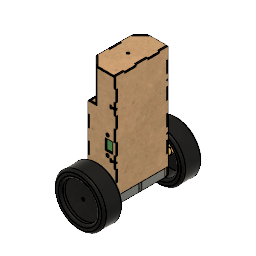
yabr6 (Autodesk Fusion 360 design; units mm, degrees)
Autodesk Fusion 360 part; units mm, degrees
note: some values were not read from the file. Chosen so that the rebuilt part matches the saved one: which bodies a step acts on. Set by a fixed rule: which sketch regions a step uses.
sketch "Sketch1" plane through (0, 0, 0) normal (0, 0, 1) x (1, 0, 0) in component "Steppers"
  line L0 (-16.6565, 21.25) -> (16.6565, 21.25)
  line L1 (21.25, 16.6565) -> (21.25, -16.6565)
  line L2 (16.6565, -21.25) -> (-16.6565, -21.25)
  line L3 (-21.25, -16.6565) -> (-21.25, 16.6565)
  circle A0 centre (-15.5, 15.5) radius 1.5
  circle A1 centre (15.5, 15.5) radius 1.5
  circle A2 centre (15.5, -15.5) radius 1.5
  circle A3 centre (-15.5, -15.5) radius 1.5
  circle A4 centre (0, 0) radius 2.5
  circle A5 centre (0, 0) radius 11.25
  arc A6 (-16.6565, 21.25) -> (-21.25, 16.6565) centre (0, 0) ccw
  arc A7 (-21.25, -16.6565) -> (-16.6565, -21.25) centre (0, 0) ccw
  arc A8 (16.6565, -21.25) -> (21.25, -16.6565) centre (0, 0) ccw
  arc A9 (21.25, 16.6565) -> (16.6565, 21.25) centre (0, 0) ccw
  dimension "d3" = 21.25
  dimension "d4" = 21.25
  dimension "d5" = 3
  dimension "d6" = 3
  dimension "d7" = 3
  dimension "d8" = 3
  dimension "d9" = 15.5
  dimension "d10" = 15.5
  dimension "d11" = 15.5
  dimension "d12" = 15.5
  dimension "d13" = 15.5
  dimension "d14" = 15.5
  dimension "d15" = 15.5
  dimension "d16" = 15.5
  dimension "d17" = 5
  dimension "d18" = 22.5
  dimension "d28" = 42.5
  dimension "d29" = 42.5
  dimension "d30" = 27
  dimension "d31" = 27
  dimension "d32" = 27
  dimension "d33" = 27
  measures "d3" distance of A4.centre L3
  measures "d4" distance of A4.centre L0
  measures "d5" diameter of A0
  measures "d6" diameter of A1
  measures "d7" diameter of A2
  measures "d8" diameter of A3
  measures "d9" distance of A4.centre
  measures "d10" distance of A4.centre
  measures "d11" distance of A4.centre
  measures "d12" distance of A4.centre
  measures "d13" distance of A4.centre
  measures "d14" distance of A4.centre
  measures "d15" distance of A4.centre
  measures "d16" distance of A4.centre
  measures "d17" diameter of A4
  measures "d18" diameter of A5
  measures "d28" distance of L1 L3
  measures "d29" distance of L0 L2
  measures "d30" radius of A6
  measures "d31" radius of A7
  measures "d32" radius of A8
  measures "d33" radius of A9
extrude "Extrude1" add sketch "Sketch1" along normal mid plane 85 contours L0 L1 L2 L3 A6 A7 A8 A9 | A4 | A5 makes body 1 in component "Steppers"
extrude "Extrude2" add sketch "Sketch1" along normal mid plane 90 contours A4 | A5 bodies 1 in component "Steppers"
extrude "Extrude3" add sketch "Sketch1" along normal mid plane 134 contours A4 bodies 1 in component "Steppers"
extrude "Extrude4" cut sketch "Sketch1" along normal mid plane 5 contours L0 L1 L2 L3 A6 A7 A8 A9 | A0 | A1 | A2 | A3 | A4 | A5 bodies 1 makes body 2 at (4.8001, -4.8266, 2.5) in component "Steppers"
sketch "Sketch1 (2)" plane through (0, 0, 42.5) normal (0, 0, 1) x (1, 0, 0) in component "MDF"
  circle A0 centre (0, 0) radius 11.25
  circle A1 centre (-15.5, -15.5) radius 1.5
  circle A2 centre (15.5, -15.5) radius 1.5
  circle A3 centre (15.5, 15.5) radius 1.5
  circle A4 centre (-15.5, 15.5) radius 1.5
  arc A5 (16.6565, -21.25) -> (21.25, -16.6565) centre (0, 0) ccw
  line L0 (21.25, -16.6565) -> (21.25, 16.6565)
  arc A6 (21.25, 16.6565) -> (16.6565, 21.25) centre (0, 0) ccw
  line L1 (16.6565, 21.25) -> (-16.6565, 21.25)
  arc A7 (-16.6565, 21.25) -> (-21.25, 16.6565) centre (0, 0) ccw
  line L2 (-21.25, 16.6565) -> (-21.25, -16.6565)
  arc A8 (-21.25, -16.6565) -> (-16.6565, -21.25) centre (0, 0) ccw
  line L3 (-16.6565, -21.25) -> (16.6565, -21.25)
  line L4 (-24.25, -11.8717) -> (-24.25, 120)
  line L5 (-24.25, 120) -> (24.25, 120)
  line L6 (24.25, 120) -> (24.25, -11.8717)
  arc A9 (-24.25, -11.8717) -> (24.25, -11.8717) centre (0, 0) ccw
  dimension "d37" = 120
  dimension "d38" = 3
  dimension "d39" = 3
  dimension "d41" = 27
  measures "d38" distance of L2 L4
  measures "d39" distance of L0 L6
  measures "d41" radius of A9
extrude "Extrude1'" add sketch "Sketch1 (2)" along normal blind 3 separate body makes body 3 in component "MDF"
copy_body "CopyPasteBodies1" bodies 3 makes body 4 in component "MDF"
move_body "Move1" bodies 4 to x (1, 0, 0) y (0, 1, 0) z (0, 0, 1) at (0, 0, -88) in component "MDF"
sketch "Sketch1 (3)" plane through (0, 0, 45) normal (0, 0, 1) x (1, 0, 0) in component "Wheels"
  circle A0 centre (0, 0) radius 2.5
  circle A1 centre (0, 0) radius 11.25
  circle A2 centre (0, 0) radius 5.5
  dimension "d47" = 11
  measures "d47" diameter of A2
extrude "Extrude1''" add sketch "Sketch1 (3)" along normal blind 24 from surface at 0.5 separate body contours A2 makes body 5 in component "Wheels"
sketch "Sketch2" plane through (0, 0, 69.5) normal (0, 0, 1) x (1, 0, 0) in component "Wheels"
  circle A0 centre (0, 0) radius 2.5
  circle A1 centre (0, 0) radius 5.5
  line L0 (-3.4641, 6) -> (-6.9282, 0)
  line L1 (-6.9282, 0) -> (-3.4641, -6)
  line L2 (-3.4641, -6) -> (3.4641, -6)
  line L3 (3.4641, -6) -> (6.9282, 0)
  line L4 (6.9282, 0) -> (3.4641, 6)
  line L5 (3.4641, 6) -> (-3.4641, 6)
  dimension "d52" = 6
  measures "d52" distance of A0.centre L5
extrude "Extrude2'" add sketch "Sketch2" along normal blind 6 contours A1 | L0 L1 L2 L3 L4 L5 bodies 5 in component "Wheels"
sketch "Sketch3" plane through (0, 0, 75.5) normal (0, 0, 1) x (1, 0, 0) in component "Wheels"
  circle A0 centre (0, 0) radius 2.5
  line L0 (3.4641, 6) -> (-3.4641, 6)
  line L1 (-3.4641, 6) -> (-6.9282, 0)
  line L2 (-6.9282, 0) -> (-3.4641, -6)
  line L3 (-3.4641, -6) -> (3.4641, -6)
  line L4 (3.4641, -6) -> (6.9282, 0)
  line L5 (6.9282, 0) -> (3.4641, 6)
  circle A1 centre (0, 0) radius 44
  dimension "d56" = 88
  measures "d56" diameter of A1
extrude "Extrude3'" add sketch "Sketch3" along normal blind 2 separate body contours L0 L1 L2 L3 L4 L5 | A1 makes body 6 in component "Wheels"
sketch "Sketch4" plane through (0, 0, 77.5) normal (0, 0, 1) x (1, 0, 0) in component "Wheels"
  circle A0 centre (0, 0) radius 2.5
  circle A1 centre (0, 0) radius 44
  circle A2 centre (0, 0) radius 31
  dimension "d61" = 62
  measures "d61" diameter of A2
extrude "Extrude4'" add sketch "Sketch4" along normal blind 8 and the other way blind 26 contours A1 bodies 6 in component "Wheels"
fillet "Fillet1" radius 4 4 edges at (-28.9021, 11.2101, 85.5) (-41.0224, -15.9111, 85.5) (-41.0224, 15.9111, 51.5) (-28.9021, -11.2101, 51.5) on bodies 6 in component "Wheels"
copy_body "CopyPasteBodies1'" bodies 5 6 makes body 7 makes body 8 in component "Wheels"
move_body "Move1'" bodies 7 8 to x (-1, 0, 0) y (0, 1, 0) z (0, 0, -1) at (0, 0, 0) in component "Wheels"
sketch "Sketch2 (2)" plane through (24.25, 0, 0) normal (1, 0, 0) x (0, 0, -1) in component "MDF"
  line L0 (0, 0) -> (-45.5, 0)
  line L1 (0, 0) -> (45.5, 0)
  line L2 (-45.5, 60) -> (-42.5, 60)
  line L3 (-42.5, 60) -> (-42.5, 80)
  line L4 (-42.5, 80) -> (-45.5, 80)
  line L5 (-45.5, 80) -> (-45.5, 100)
  line L6 (-45.5, 100) -> (-42.5, 100)
  line L7 (-42.5, 100) -> (-42.5, 120)
  line L8 (-42.5, 120) -> (-45.5, 120)
  line L9 (-45.5, 120) -> (-45.5, 140)
  line L10 (-45.5, 140) -> (-42.5, 140)
  line L11 (-42.5, 140) -> (-42.5, 160)
  line L12 (-42.5, 160) -> (-45.5, 160)
  line L13 (-45.5, 160) -> (-45.5, 180)
  line L14 (45.5, 180) -> (45.5, 160)
  line L15 (45.5, 160) -> (42.5, 160)
  line L16 (42.5, 160) -> (42.5, 140)
  line L17 (42.5, 140) -> (45.5, 140)
  line L18 (45.5, 140) -> (45.5, 120)
  line L19 (45.5, 120) -> (42.5, 120)
  line L20 (42.5, 120) -> (42.5, 100)
  line L21 (42.5, 100) -> (45.5, 100)
  line L22 (45.5, 100) -> (45.5, 80)
  line L23 (45.5, 80) -> (42.5, 80)
  line L24 (42.5, 80) -> (42.5, 60)
  line L25 (42.5, 60) -> (45.5, 60)
  line L26 (45.5, 180) -> (30, 180)
  line L27 (30, 180) -> (30, 177)
  line L28 (30, 177) -> (10, 177)
  line L29 (10, 177) -> (10, 180)
  line L30 (10, 180) -> (-10, 180)
  line L31 (-10, 180) -> (-10, 177)
  line L32 (-10, 177) -> (-30, 177)
  line L33 (-30, 177) -> (-30, 180)
  line L34 (-30, 180) -> (-45.5, 180)
  line L35 (0, 0) -> (0, 242.7962) construction
  line L36 (45.5, 60) -> (45.5, 40)
  line L37 (45.5, 40) -> (42.5, 40)
  line L38 (42.5, 40) -> (42.5, 20)
  line L39 (42.5, 20) -> (45.5, 20)
  line L40 (45.5, 20) -> (45.5, 0)
  line L41 (-45.5, 60) -> (-45.5, 40)
  line L42 (-45.5, 40) -> (-42.5, 40)
  line L43 (-42.5, 40) -> (-42.5, 20)
  line L44 (-42.5, 20) -> (-45.5, 20)
  line L45 (-45.5, 20) -> (-45.5, 0)
  dimension "d69" = 3
  dimension "d70" = 20
  dimension "d71" = 3
  dimension "d72" = 20
  dimension "d73" = 3
  dimension "d74" = 20
  dimension "d75" = 3
  dimension "d76" = 20
  dimension "d77" = 3
  dimension "d78" = 20
  dimension "d79" = 3
  dimension "d80" = 20
  dimension "d82" = 3
  dimension "d83" = 20
  dimension "d84" = 3
  dimension "d85" = 20
  dimension "d86" = 3
  dimension "d87" = 20
  dimension "d88" = 3
  dimension "d89" = 20
  dimension "d90" = 3
  dimension "d91" = 20
  dimension "d92" = 3
  dimension "d96" = 20
  dimension "d97" = 10
  dimension "d98" = 10
  dimension "d99" = 3
  dimension "d100" = 20
  dimension "d101" = 3
  dimension "d102" = 3
  dimension "d103" = 20
  dimension "d104" = 3
  dimension "d105" = 3
  dimension "d106" = 20
  dimension "d107" = 20
  dimension "d108" = 20
  dimension "d109" = 3
  dimension "d110" = 3
  dimension "d111" = 20
  dimension "d112" = 20
  dimension "d113" = 20
  measures "d97" distance of L29 L35
  measures "d98" distance of L31 L35
  measures "d100" distance of L0.start
  measures "d103" distance of L0.start
  measures "d106" distance of L0.start
  measures "d111" distance of L0.start
  measures "d112" distance of L0.start
extrude "Extrude2''" add sketch "Sketch2 (2)" against normal blind 3 separate body makes body 9 in component "MDF"
combine "Combine1" operation cut target body 3 tool bodies 9 keep tools in component "MDF"
combine "Combine2" operation cut target body 4 tool bodies 9 keep tools in component "MDF"
sketch "Sketch16" plane through (0, 120, 0) normal (0, 1, 0) x (-1, 0, 0) in component "MDF"
  line L0 (-24.25, -45.5) -> (24.25, -45.5)
  line L1 (24.25, -45.5) -> (24.25, -42.5)
  line L2 (24.25, -42.5) -> (-24.25, -42.5)
  line L3 (-24.25, -42.5) -> (-24.25, -45.5)
  line L4 (24.25, -45.5) -> (-75.4847, -45.5) construction
  line L5 (24.25, -45.5) -> (24.25, 30) construction
  line L6 (24.25, -42.5) -> (-74.737, -42.5) construction
  line L7 (21.25, -45.5) -> (21.25, 30) construction
  line L8 (21.25, -30.2972) -> (9.0472, -42.5)
  line L9 (24.25, -31.5398) -> (10.2898, -45.5)
  line L10 (10.2898, -45.5) -> (8.1685, -43.3787)
  line L11 (9.0472, -42.5) -> (8.1685, -43.3787)
  line L12 (24.25, -31.5398) -> (22.1287, -29.4185)
  line L13 (21.25, -30.2972) -> (22.1287, -29.4185)
  line L14 (8.1685, -43.3787) -> (8.1685, -42.5) construction
  line L15 (22.1287, -29.4185) -> (21.25, -29.4185) construction
  line L16 (0, 0) -> (81.4572, 0) construction
  line L17 (21.25, 30.2972) -> (9.0472, 42.5)
  line L18 (9.0472, 42.5) -> (8.1685, 43.3787)
  line L19 (10.2898, 45.5) -> (8.1685, 43.3787)
  line L20 (24.25, 31.5398) -> (10.2898, 45.5)
  line L21 (24.25, 31.5398) -> (22.1287, 29.4185)
  line L22 (21.25, 30.2972) -> (22.1287, 29.4185)
  dimension "d248" = 3
  dimension "d249" = 3
  dimension "d251" = 45
  dimension "d253" = 3
  dimension "d254" = 18.5
  measures "d248" distance of L4 L6
  measures "d249" distance of L5 L7
  measures "d251" angle of L6 L8
  measures "d253" distance of L8 L9
  measures "d254" distance of L16.start
extrude "Extrude11" add sketch "Sketch16" along normal blind 60 separate body contours L2 L9 L10 L11 | L2 L8 L9 L12 L13 | L17 L18 L19 L20 L21 L22 makes body 10 at (-12.8219, 140, -38.7253) makes body 11 at (-17.4753, 140, 34.0719) in component "MDF"
sketch "Sketch17" plane through (-27.8949, 0, -27.8949) normal (-0.707107, 0, -0.707107) x (-0.707107, 0, 0.707107) in component "MDF"
  line L0 (-24.8973, 120) -> (-5.1547, 120)
  line L1 (-5.1547, 120) -> (-5.1547, 180)
  line L2 (-5.1547, 180) -> (-24.8973, 180)
  line L3 (-24.8973, 180) -> (-24.8973, 120)
  line L4 (-24.8973, 150) -> (-5.1547, 150) construction
  line L5 (-15.026, 180) -> (-15.026, 120) construction
  circle A0 centre (-15.026, 162.7) radius 8.1
  circle A1 centre (-15.026, 137.3) radius 8.1
  dimension "d257" = 12.7
  dimension "d258" = 12.7
  dimension "d259" = 16.2
  dimension "d260" = 16.2
  measures "d257" distance of L4
  measures "d258" distance of L4
  measures "d259" diameter of A0
  measures "d260" diameter of A1
extrude "Extrude12" cut sketch "Sketch17" against normal blind 3 contours A0 | A1 bodies 10 in component "MDF"
sketch "Sketch18" plane through (-27.8949, 0, 27.8949) normal (-0.707107, 0, 0.707107) x (0.707107, 0, 0.707107) in component "MDF"
  line L0 (5.1547, 120) -> (24.8973, 120)
  line L1 (24.8973, 120) -> (24.8973, 180)
  line L2 (24.8973, 180) -> (5.1547, 180)
  line L3 (5.1547, 180) -> (5.1547, 120)
  line L4 (15.026, 180) -> (15.026, 120) construction
  line L5 (24.8973, 150) -> (5.1547, 150) construction
  circle A0 centre (15.026, 162.7) radius 8.1
  circle A1 centre (15.026, 137.3) radius 8.1
  dimension "d263" = 12.7
  dimension "d264" = 12.7
  dimension "d265" = 16.2
  dimension "d266" = 16.2
  measures "d263" distance of L5
  measures "d264" distance of L5
  measures "d265" diameter of A0
  measures "d266" diameter of A1
extrude "Extrude13" cut sketch "Sketch18" against normal blind 3 contours A0 | A1 bodies 11 in component "MDF"
sketch "Sketch19" plane through (-24.25, 0, 0) normal (-1, 0, 0) x (0, 0, 1) in component "MDF"
  line L0 (-45.5, 0) -> (-45.5, 20)
  line L1 (-42.5, 20) -> (-42.5, 40)
  line L2 (-45.5, 40) -> (-45.5, 60)
  line L3 (-42.5, 60) -> (-42.5, 80)
  line L4 (-45.5, 80) -> (-45.5, 100)
  line L5 (-10, 177) -> (-10, 180)
  line L6 (-10, 180) -> (10, 180)
  line L7 (10, 180) -> (10, 177)
  line L8 (10, 177) -> (29.4185, 177)
  line L9 (29.4185, 177) -> (29.4185, 120)
  line L10 (29.4185, 120) -> (42.5, 120)
  line L11 (42.5, 120) -> (42.5, 100)
  line L12 (42.5, 100) -> (45.5, 100)
  line L13 (45.5, 100) -> (45.5, 80)
  line L14 (45.5, 80) -> (42.5, 80)
  line L15 (42.5, 80) -> (42.5, 60)
  line L16 (42.5, 60) -> (45.5, 60)
  line L17 (45.5, 60) -> (45.5, 40)
  line L18 (45.5, 40) -> (42.5, 40)
  line L19 (42.5, 40) -> (42.5, 20)
  line L20 (42.5, 20) -> (45.5, 20)
  line L21 (45.5, 20) -> (45.5, 0)
  line L22 (-45.5, 20) -> (-42.5, 20)
  line L23 (-42.5, 40) -> (-45.5, 40)
  line L24 (-45.5, 60) -> (-42.5, 60)
  line L25 (-42.5, 80) -> (-45.5, 80)
  line L26 (-45.5, 100) -> (-42.5, 100)
  line L27 (-42.5, 100) -> (-42.5, 120)
  line L28 (-42.5, 120) -> (-29.4185, 120)
  line L29 (-29.4185, 120) -> (-29.4185, 177)
  line L30 (-29.4185, 177) -> (-10, 177)
  line L31 (-45.5, 0) -> (45.5, 0)
extrude "Extrude14" add sketch "Sketch19" against normal blind 3 separate body makes body 12 in component "MDF"
combine "Combine5" operation cut target body 4 tool bodies 12 keep tools in component "MDF"
combine "Combine6" operation cut target body 3 tool bodies 12 keep tools in component "MDF"
sketch "Sketch20" plane through (0, 180, 0) normal (0, 1, 0) x (-1, 0, 0) in component "MDF"
  line L0 (-24.25, -10) -> (-21.25, -10)
  line L1 (-21.25, -10) -> (-21.25, 10)
  line L2 (-21.25, 10) -> (-24.25, 10)
  line L3 (-21.25, 45.5) -> (-21.25, 30)
  line L4 (-24.25, 30) -> (-24.25, 10)
  line L5 (-21.25, 10) -> (-21.25, -10)
  line L6 (-24.25, -10) -> (-24.25, -30)
  line L7 (-24.25, -30) -> (-21.25, -30)
  line L8 (-21.25, -45.5) -> (8.1685, -45.5)
  line L9 (8.1685, -45.5) -> (8.1685, -43.3787)
  line L10 (22.1287, -29.4185) -> (8.1685, -43.3787)
  line L11 (8.1685, -43.3787) -> (22.1287, -29.4185)
  line L12 (24.25, -29.4185) -> (24.25, -10)
  line L13 (21.25, -10) -> (21.25, 10)
  line L14 (24.25, 10) -> (24.25, 29.4185)
  line L15 (8.1685, 43.3787) -> (22.1287, 29.4185)
  line L16 (22.1287, 29.4185) -> (8.1685, 43.3787)
  line L17 (8.1685, 43.3787) -> (8.1685, 45.5)
  line L18 (8.1685, 45.5) -> (-21.25, 45.5)
  line L19 (-21.25, -45.5) -> (-21.25, -30)
  line L20 (-21.25, -10) -> (-24.25, -10)
  line L21 (-24.25, 10) -> (-21.25, 10)
  line L22 (-21.25, 30) -> (-24.25, 30)
  line L23 (22.1287, 29.4185) -> (24.25, 29.4185)
  line L24 (24.25, 10) -> (21.25, 10)
  line L25 (24.25, -10) -> (21.25, -10)
  line L26 (24.25, -29.4185) -> (22.1287, -29.4185)
extrude "Extrude15" add sketch "Sketch20" against normal blind 3 separate body makes body 13 in component "MDF"
sketch "Sketch21" plane through (0, 0, -45.5) normal (0, 0, -1) x (-1, 0, 0) in component "MDF"
  circle A0 centre (15.5, 15.5) radius 1.5
  circle A1 centre (-15.5, 15.5) radius 1.5
  circle A2 centre (0, 0) radius 11.25
  circle A3 centre (-15.5, -15.5) radius 1.5
  circle A4 centre (15.5, -15.5) radius 1.5
  line L0 (24.25, 0) -> (21.25, 0)
  line L1 (21.25, 0) -> (21.25, 20)
  line L2 (21.25, 20) -> (24.25, 20)
  line L3 (24.25, 20) -> (24.25, 40)
  line L4 (24.25, 40) -> (21.25, 40)
  line L5 (21.25, 40) -> (21.25, 60)
  line L6 (21.25, 60) -> (24.25, 60)
  line L7 (24.25, 60) -> (24.25, 80)
  line L8 (24.25, 80) -> (21.25, 80)
  line L9 (21.25, 80) -> (21.25, 100)
  line L10 (21.25, 100) -> (24.25, 100)
  line L11 (24.25, 100) -> (24.25, 120)
  line L12 (24.25, 120) -> (-24.25, 120)
  line L13 (-24.25, 120) -> (-24.25, 100)
  line L14 (-24.25, 100) -> (-21.25, 100)
  line L15 (-21.25, 100) -> (-21.25, 80)
  line L16 (-21.25, 80) -> (-24.25, 80)
  line L17 (-24.25, 80) -> (-24.25, 60)
  line L18 (-24.25, 60) -> (-21.25, 60)
  line L19 (-21.25, 60) -> (-21.25, 40)
  line L20 (-21.25, 40) -> (-24.25, 40)
  line L21 (-24.25, 40) -> (-24.25, 20)
  line L22 (-24.25, 20) -> (-21.25, 20)
  line L23 (-21.25, 20) -> (-21.25, 0)
  line L24 (-21.25, 0) -> (-24.25, 0)
  line L25 (-24.25, 0) -> (-24.25, -11.8717)
  arc A5 (-24.25, -11.8717) -> (24.25, -11.8717) centre (0, 0) ccw
  line L26 (24.25, -11.8717) -> (24.25, 0)
  line L27 (-21.25, 120) -> (-21.25, 140)
  line L28 (-21.25, 140) -> (-24.25, 140)
  line L29 (-24.25, 140) -> (-24.25, 160)
  line L30 (-24.25, 160) -> (-21.25, 160)
  line L31 (-21.25, 160) -> (-21.25, 177)
  line L32 (-21.25, 177) -> (8.1685, 177)
  line L33 (8.1685, 177) -> (8.1685, 120)
extrude "Extrude16" add sketch "Sketch21" against normal blind 3 contours L12 L27 L28 L29 L30 L31 L32 L33 bodies 4 in component "MDF"
sketch "Sketch22" plane through (0, 0, 45.5) normal (0, 0, 1) x (1, 0, 0) in component "MDF"
  line L0 (-21.25, 0) -> (-24.25, 0)
  line L1 (-24.25, 0) -> (-24.25, -11.8717)
  arc A0 (-24.25, -11.8717) -> (24.25, -11.8717) centre (0, 0) ccw
  line L2 (24.25, -11.8717) -> (24.25, 0)
  line L3 (24.25, 0) -> (21.25, 0)
  line L4 (21.25, 0) -> (21.25, 20)
  line L5 (21.25, 20) -> (24.25, 20)
  line L6 (24.25, 20) -> (24.25, 40)
  line L7 (24.25, 40) -> (21.25, 40)
  line L8 (21.25, 40) -> (21.25, 60)
  line L9 (21.25, 60) -> (24.25, 60)
  line L10 (24.25, 60) -> (24.25, 80)
  line L11 (24.25, 80) -> (21.25, 80)
  line L12 (21.25, 80) -> (21.25, 100)
  line L13 (21.25, 100) -> (24.25, 100)
  line L14 (24.25, 100) -> (24.25, 120)
  line L15 (24.25, 120) -> (-24.25, 120)
  line L16 (-24.25, 120) -> (-24.25, 100)
  line L17 (-24.25, 100) -> (-21.25, 100)
  line L18 (-21.25, 100) -> (-21.25, 80)
  line L19 (-21.25, 80) -> (-24.25, 80)
  line L20 (-24.25, 80) -> (-24.25, 60)
  line L21 (-24.25, 60) -> (-21.25, 60)
  line L22 (-21.25, 60) -> (-21.25, 40)
  line L23 (-21.25, 40) -> (-24.25, 40)
  line L24 (-24.25, 40) -> (-24.25, 20)
  line L25 (-24.25, 20) -> (-21.25, 20)
  line L26 (-21.25, 20) -> (-21.25, 0)
  circle A1 centre (-15.5, 15.5) radius 1.5
  circle A2 centre (15.5, 15.5) radius 1.5
  circle A3 centre (0, 0) radius 11.25
  circle A4 centre (15.5, -15.5) radius 1.5
  circle A5 centre (-15.5, -15.5) radius 1.5
  line L27 (21.25, 120) -> (21.25, 140)
  line L28 (21.25, 140) -> (24.25, 140)
  line L29 (24.25, 140) -> (24.25, 160)
  line L30 (24.25, 160) -> (21.25, 160)
  line L31 (21.25, 160) -> (21.25, 177)
  line L32 (21.25, 177) -> (-8.1685, 177)
  line L33 (-8.1685, 177) -> (-8.1685, 120)
extrude "Extrude17" add sketch "Sketch22" against normal blind 3 contours L15 L27 L28 L29 L30 L31 L32 L33 bodies 3 in component "MDF"
sketch "Sketch23" plane through (-24.25, 0, 0) normal (-1, 0, 0) x (0, 0, 1) in component "MDF"
  line L0 (-45.5, 20) -> (-45.5, 0)
  line L1 (-45.5, 0) -> (45.5, 0)
  line L2 (45.5, 0) -> (45.5, 20)
  line L3 (45.5, 20) -> (42.5, 20)
  line L4 (42.5, 20) -> (42.5, 40)
  line L5 (42.5, 40) -> (45.5, 40)
  line L6 (45.5, 40) -> (45.5, 60)
  line L7 (45.5, 60) -> (42.5, 60)
  line L8 (42.5, 60) -> (42.5, 80)
  line L9 (42.5, 80) -> (45.5, 80)
  line L10 (45.5, 80) -> (45.5, 100)
  line L11 (45.5, 100) -> (42.5, 100)
  line L12 (42.5, 100) -> (42.5, 120)
  line L13 (42.5, 120) -> (29.4185, 120)
  line L14 (29.4185, 120) -> (29.4185, 177)
  line L15 (29.4185, 177) -> (10, 177)
  line L16 (10, 177) -> (10, 180)
  line L17 (10, 180) -> (-10, 180)
  line L18 (-10, 180) -> (-10, 177)
  line L19 (-10, 177) -> (-29.4185, 177)
  line L20 (-29.4185, 177) -> (-29.4185, 120)
  line L21 (-29.4185, 120) -> (-42.5, 120)
  line L22 (-42.5, 120) -> (-42.5, 100)
  line L23 (-42.5, 100) -> (-45.5, 100)
  line L24 (-45.5, 100) -> (-45.5, 80)
  line L25 (-45.5, 80) -> (-42.5, 80)
  line L26 (-42.5, 80) -> (-42.5, 60)
  line L27 (-42.5, 60) -> (-45.5, 60)
  line L28 (-45.5, 60) -> (-45.5, 40)
  line L29 (-45.5, 40) -> (-42.5, 40)
  line L30 (-42.5, 40) -> (-42.5, 20)
  line L31 (-42.5, 20) -> (-45.5, 20)
  line L32 (0, 180) -> (0, 120) construction
  line L33 (-29.4185, 120) -> (29.4185, 120) construction
  line L34 (0, 150) -> (20, 150) construction
  line L35 (0, 150) -> (-20, 150) construction
  circle A0 centre (0, 162.7) radius 8.1
  circle A1 centre (0, 137.3) radius 8.1
  dimension "d277" = 12.7
  dimension "d278" = 12.7
  dimension "d279" = 16.2
  dimension "d280" = 16.2
  measures "d278" distance of L34 origin
  measures "d279" diameter of A0
  measures "d280" diameter of A1
extrude "Extrude18" cut sketch "Sketch23" against normal blind 3 contours A0 | A1 bodies 12 in component "MDF"
sketch "Sketch1 (4)" plane through (0, 0, 0) normal (0, 1, 0) x (1, 0, 0) in component "ground plane"
  line L0 (-5000, 5000) -> (5000, 5000)
  line L1 (5000, 5000) -> (5000, -5000)
  line L2 (5000, -5000) -> (-5000, -5000)
  line L3 (-5000, -5000) -> (-5000, 5000)
extrude "Extrude1'''" add sketch "Sketch1 (4)" against normal blind 50 from surface at -44 separate body makes body 14 in component "ground plane"
sketch "Sketch1 (5)" plane through (21.25, 0, 0) normal (-1, 0, 0) x (0, 0, 1) in component "pcb"
  line L0 (45.5, 40) -> (45.5, 60)
  line L1 (45.5, 60) -> (42.5, 60)
  line L2 (42.5, 60) -> (42.5, 80)
  line L3 (42.5, 80) -> (45.5, 80)
  line L4 (45.5, 80) -> (45.5, 100)
  line L5 (45.5, 100) -> (42.5, 100)
  line L6 (42.5, 100) -> (42.5, 120)
  line L7 (42.5, 120) -> (45.5, 120)
  line L8 (45.5, 120) -> (45.5, 140)
  line L9 (45.5, 140) -> (42.5, 140)
  line L10 (42.5, 140) -> (42.5, 160)
  line L11 (42.5, 160) -> (45.5, 160)
  line L12 (45.5, 160) -> (45.5, 180)
  line L13 (45.5, 180) -> (30, 180)
  line L14 (30, 180) -> (30, 177)
  line L15 (30, 177) -> (10, 177)
  line L16 (10, 177) -> (10, 180)
  line L17 (10, 180) -> (-10, 180)
  line L18 (-10, 180) -> (-10, 177)
  line L19 (-10, 177) -> (-30, 177)
  line L20 (-30, 177) -> (-30, 180)
  line L21 (-30, 180) -> (-45.5, 180)
  line L22 (-45.5, 180) -> (-45.5, 160)
  line L23 (-45.5, 160) -> (-42.5, 160)
  line L24 (-42.5, 160) -> (-42.5, 140)
  line L25 (-42.5, 140) -> (-45.5, 140)
  line L26 (-45.5, 140) -> (-45.5, 120)
  line L27 (-45.5, 120) -> (-42.5, 120)
  line L28 (-42.5, 120) -> (-42.5, 100)
  line L29 (-42.5, 100) -> (-45.5, 100)
  line L30 (-45.5, 100) -> (-45.5, 80)
  line L31 (-45.5, 80) -> (-42.5, 80)
  line L32 (-42.5, 80) -> (-42.5, 60)
  line L33 (-42.5, 60) -> (-45.5, 60)
  line L34 (-45.5, 60) -> (-45.5, 40)
  line L35 (-45.5, 40) -> (-42.5, 40)
  line L36 (-42.5, 40) -> (-42.5, 20)
  line L37 (-42.5, 20) -> (-45.5, 20)
  line L38 (-45.5, 20) -> (-45.5, 0)
  line L39 (-45.5, 0) -> (45.5, 0)
  line L40 (45.5, 0) -> (45.5, 20)
  line L41 (45.5, 20) -> (42.5, 20)
  line L42 (42.5, 20) -> (42.5, 40)
  line L43 (42.5, 40) -> (45.5, 40)
  line L44 (-39.37, 26) -> (-39.37, 86.96)
  line L45 (-39.37, 86.96) -> (39.37, 86.96)
  line L46 (39.37, 86.96) -> (39.37, 26)
  line L47 (-39.37, 26) -> (39.37, 26)
  line L48 (-39.37, 56.48) -> (39.37, 56.48) construction
  line L49 (0, 86.96) -> (0, 26) construction
  circle A0 centre (-31.75, 79.34) radius 1.5
  circle A1 centre (31.75, 79.34) radius 1.5
  circle A2 centre (26.67, 38.7) radius 1.5
  circle A3 centre (-26.67, 38.7) radius 1.5
  dimension "d289" = 78.74
  dimension "d290" = 26
  dimension "d291" = 39.37
  dimension "d295" = 3
  dimension "d296" = 3
  dimension "d297" = 3
  dimension "d298" = 3
  dimension "d315" = 12.7
  dimension "d316" = 12.7
  dimension "d317" = 12.7
  dimension "d318" = 12.7
  dimension "d319" = 7.62
  dimension "d320" = 7.62
  dimension "d321" = 60.96
  dimension "d323" = 53.34
  dimension "d324" = 53.34
  measures "d295" diameter of A0
  measures "d296" diameter of A1
  measures "d297" diameter of A3
  measures "d298" diameter of A2
  measures "d321" distance of L45 L47
extrude "Extrude1''''" add sketch "Sketch1 (5)" along normal blind 1 from surface at 40 separate body contours L44 L45 L46 L47 makes body 15 in component "pcb"
sketch "Sketch25" plane through (-18.75, 0, 0) normal (1, 0, 0) x (0, 0, -1) in component "MDF"
  circle A0 centre (-26.67, 38.7) radius 1.5
  circle A1 centre (26.67, 38.7) radius 1.5
  circle A2 centre (-31.75, 79.34) radius 1.5
  circle A3 centre (31.75, 79.34) radius 1.5
  line L0 (39.37, 26) -> (39.37, 86.96)
  line L1 (39.37, 86.96) -> (-39.37, 86.96)
  line L2 (-39.37, 86.96) -> (-39.37, 26)
  line L3 (-39.37, 26) -> (39.37, 26)
extrude "Extrude19" cut sketch "Sketch25" against normal blind 10 contours A0 | A1 | A2 | A3 bodies 12 in component "MDF"
sketch "Sketch1 (6)" plane through (24.25, 0, 0) normal (1, 0, 0) x (0, 0, -1)
  line L0 (-45.5, 60) -> (-45.5, 40)
  line L1 (-45.5, 40) -> (-42.5, 40)
  line L2 (-42.5, 40) -> (-42.5, 20)
  line L3 (-42.5, 20) -> (-45.5, 20)
  line L4 (-45.5, 20) -> (-45.5, 0)
  line L5 (-45.5, 0) -> (45.5, 0)
  line L6 (45.5, 0) -> (45.5, 20)
  line L7 (45.5, 20) -> (42.5, 20)
  line L8 (42.5, 20) -> (42.5, 40)
  line L9 (42.5, 40) -> (45.5, 40)
  line L10 (45.5, 40) -> (45.5, 60)
  line L11 (45.5, 60) -> (42.5, 60)
  line L12 (42.5, 60) -> (42.5, 80)
  line L13 (42.5, 80) -> (45.5, 80)
  line L14 (45.5, 80) -> (45.5, 100)
  line L15 (45.5, 100) -> (42.5, 100)
  line L16 (42.5, 100) -> (42.5, 120)
  line L17 (42.5, 120) -> (45.5, 120)
  line L18 (45.5, 120) -> (45.5, 140)
  line L19 (45.5, 140) -> (42.5, 140)
  line L20 (42.5, 140) -> (42.5, 160)
  line L21 (42.5, 160) -> (45.5, 160)
  line L22 (45.5, 160) -> (45.5, 180)
  line L23 (45.5, 180) -> (30, 180)
  line L24 (30, 180) -> (30, 177)
  line L25 (30, 177) -> (10, 177)
  line L26 (10, 177) -> (10, 180)
  line L27 (10, 180) -> (-10, 180)
  line L28 (-10, 180) -> (-10, 177)
  line L29 (-10, 177) -> (-30, 177)
  line L30 (-30, 177) -> (-30, 180)
  line L31 (-30, 180) -> (-45.5, 180)
  line L32 (-45.5, 180) -> (-45.5, 160)
  line L33 (-45.5, 160) -> (-42.5, 160)
  line L34 (-42.5, 160) -> (-42.5, 140)
  line L35 (-42.5, 140) -> (-45.5, 140)
  line L36 (-45.5, 140) -> (-45.5, 120)
  line L37 (-45.5, 120) -> (-42.5, 120)
  line L38 (-42.5, 120) -> (-42.5, 100)
  line L39 (-42.5, 100) -> (-45.5, 100)
  line L40 (-45.5, 100) -> (-45.5, 80)
  line L41 (-45.5, 80) -> (-42.5, 80)
  line L42 (-42.5, 80) -> (-42.5, 60)
  line L43 (-42.5, 60) -> (-45.5, 60)
  line L44 (-45.5, 60) -> (-42.5, 40) construction
  circle A0 centre (-44, 50) radius 1.5
  line L45 (45.5, 60) -> (42.5, 40) construction
  circle A1 centre (44, 50) radius 1.5
  line L46 (45.5, 140) -> (42.5, 120) construction
  circle A2 centre (44, 130) radius 1.5
  line L47 (-45.5, 140) -> (-42.5, 120) construction
  circle A3 centre (-44, 130) radius 1.5
  dimension "d327" = 3
  dimension "d328" = 3
  dimension "d329" = 3
  dimension "d330" = 3
  measures "d327" diameter of A0
  measures "d328" diameter of A1
  measures "d329" diameter of A2
  measures "d330" diameter of A3
extrude "Extrude20" cut sketch "Sketch1 (6)" against normal blind 3 contours A0 | A1 | A2 | A3 bodies 9 in component "MDF"
sketch "Sketch26" plane through (0, 0, 45.5) normal (0, 0, 1) x (1, 0, 0) in component "MDF"
  line L0 (-21.25, 0) -> (-24.25, 0)
  line L1 (-24.25, 0) -> (-24.25, -11.8717)
  arc A0 (-24.25, -11.8717) -> (24.25, -11.8717) centre (0, 0) ccw
  line L2 (24.25, -11.8717) -> (24.25, 0)
  line L3 (24.25, 0) -> (21.25, 0)
  line L4 (21.25, 0) -> (21.25, 20)
  line L5 (21.25, 20) -> (24.25, 20)
  line L6 (24.25, 20) -> (24.25, 40)
  line L7 (24.25, 40) -> (21.25, 40)
  line L8 (21.25, 40) -> (21.25, 60)
  line L9 (21.25, 60) -> (24.25, 60)
  line L10 (24.25, 60) -> (24.25, 80)
  line L11 (24.25, 80) -> (21.25, 80)
  line L12 (21.25, 80) -> (21.25, 100)
  line L13 (21.25, 100) -> (24.25, 100)
  line L14 (24.25, 100) -> (24.25, 120)
  line L15 (24.25, 120) -> (21.25, 120)
  line L16 (21.25, 120) -> (21.25, 140)
  line L17 (21.25, 140) -> (24.25, 140)
  line L18 (24.25, 140) -> (24.25, 160)
  line L19 (24.25, 160) -> (21.25, 160)
  line L20 (21.25, 160) -> (21.25, 177)
  line L21 (21.25, 177) -> (-8.1685, 177)
  line L22 (-8.1685, 177) -> (-8.1685, 120)
  line L23 (-8.1685, 120) -> (-24.25, 120)
  line L24 (-24.25, 120) -> (-24.25, 100)
  line L25 (-24.25, 100) -> (-21.25, 100)
  line L26 (-21.25, 100) -> (-21.25, 80)
  line L27 (-21.25, 80) -> (-24.25, 80)
  line L28 (-24.25, 80) -> (-24.25, 60)
  line L29 (-24.25, 60) -> (-21.25, 60)
  line L30 (-21.25, 60) -> (-21.25, 40)
  line L31 (-21.25, 40) -> (-24.25, 40)
  line L32 (-24.25, 40) -> (-24.25, 20)
  line L33 (-24.25, 20) -> (-21.25, 20)
  line L34 (-21.25, 20) -> (-21.25, 0)
  circle A1 centre (-15.5, -15.5) radius 1.5
  circle A2 centre (0, 0) radius 11.25
  circle A3 centre (15.5, -15.5) radius 1.5
  circle A4 centre (15.5, 15.5) radius 1.5
  circle A5 centre (-15.5, 15.5) radius 1.5
  line L35 (21.25, 130) -> (21.25, 131.5)
  line L36 (16.75, 131.5) -> (16.75, 132.85)
  line L37 (16.75, 132.85) -> (14.25, 132.85)
  line L38 (14.25, 132.85) -> (14.25, 127.15)
  line L39 (14.25, 127.15) -> (16.75, 127.15)
  line L40 (16.75, 127.15) -> (16.75, 128.5)
  line L41 (16.75, 128.5) -> (21.25, 128.5)
  line L42 (21.25, 130) -> (21.25, 128.5)
  line L43 (21.25, 131.5) -> (16.75, 131.5)
  line L44 (21.25, 50) -> (21.25, 51.5)
  line L45 (21.25, 50) -> (21.25, 48.5)
  line L46 (21.25, 51.5) -> (16.75, 51.5)
  line L47 (16.75, 51.5) -> (16.75, 52.85)
  line L48 (14.25, 47.15) -> (16.75, 47.15)
  line L49 (16.75, 48.5) -> (21.25, 48.5)
  line L50 (16.75, 52.85) -> (14.25, 52.85)
  line L51 (14.25, 52.85) -> (14.25, 47.15)
  line L52 (16.75, 47.15) -> (16.75, 48.5)
  dimension "d333" = 3
  dimension "d334" = 1.5
  dimension "d335" = 2.5
  dimension "d336" = 7
  dimension "d337" = 5.7
  dimension "d338" = 2.85
  dimension "d339" = 3
  dimension "d340" = 1.5
  dimension "d341" = 2.5
  dimension "d342" = 7
  dimension "d343" = 5.7
  dimension "d344" = 2.85
  measures "d333" distance of L41 L43
  measures "d336" distance of L38 A0.centre
  measures "d337" distance of L37 L39
  measures "d338" distance of A0.centre L37
  measures "d339" distance of L46 L49
  measures "d342" distance of A0.centre L51
  measures "d343" distance of L48 L50
  measures "d344" distance of A0.centre L50
extrude "Extrude21" cut sketch "Sketch26" against normal blind 200 contours L8 L44 L45 L46 L47 L48 L49 L50 L51 L52 | L16 L35 L36 L37 L38 L39 L40 L41 L42 L43 bodies 3 4 in component "MDF"
sketch "Sketch27" plane through (0, 180, 0) normal (0, 1, 0) x (-1, 0, 0) in component "MDF"
  line L0 (24.25, -10) -> (21.25, -10)
  line L1 (21.25, -10) -> (21.25, 10)
  line L2 (21.25, 10) -> (24.25, 10)
  line L3 (24.25, 10) -> (24.25, 29.4185)
  line L4 (24.25, 29.4185) -> (22.1287, 29.4185)
  line L5 (22.1287, 29.4185) -> (8.1685, 43.3787)
  line L6 (8.1685, 43.3787) -> (8.1685, 45.5)
  line L7 (8.1685, 45.5) -> (-21.25, 45.5)
  line L8 (-21.25, 45.5) -> (-21.25, 30)
  line L9 (-21.25, 30) -> (-24.25, 30)
  line L10 (-24.25, 30) -> (-24.25, 10)
  line L11 (-24.25, 10) -> (-21.25, 10)
  line L12 (-21.25, 10) -> (-21.25, -10)
  line L13 (-21.25, -10) -> (-24.25, -10)
  line L14 (-24.25, -10) -> (-24.25, -30)
  line L15 (-24.25, -30) -> (-21.25, -30)
  line L16 (-21.25, -30) -> (-21.25, -45.5)
  line L17 (-21.25, -45.5) -> (8.1685, -45.5)
  line L18 (8.1685, -45.5) -> (8.1685, -43.3787)
  line L19 (8.1685, -43.3787) -> (22.1287, -29.4185)
  line L20 (22.1287, -29.4185) -> (24.25, -29.4185)
  line L21 (24.25, -29.4185) -> (24.25, -10)
  circle A0 centre (0, 0) radius 2.5
  dimension "d350" = 5
  measures "d350" diameter of A0
extrude "Extrude23" cut sketch "Sketch27" against normal blind 3 contours A0 bodies 13 in component "MDF"
sketch "Sketch2 (3)" plane through (-21.25, 0, 0) normal (1, 0, 0) x (0, 0, -1)
  circle A0 centre (31.75, 79.34) radius 1.5
  circle A1 centre (26.67, 38.7) radius 1.5
  circle A2 centre (-31.75, 79.34) radius 1.5
  circle A3 centre (-26.67, 38.7) radius 1.5
  circle A4 centre (0, 162.7) radius 8.1
  circle A5 centre (0, 137.3) radius 8.1
  line L0 (45.5, 0) -> (45.5, 20)
  line L1 (45.5, 20) -> (42.5, 20)
  line L2 (42.5, 20) -> (42.5, 40)
  line L3 (42.5, 40) -> (45.5, 40)
  line L4 (45.5, 40) -> (45.5, 60)
  line L5 (45.5, 60) -> (42.5, 60)
  line L6 (42.5, 60) -> (42.5, 80)
  line L7 (42.5, 80) -> (45.5, 80)
  line L8 (45.5, 80) -> (45.5, 100)
  line L9 (45.5, 100) -> (42.5, 100)
  line L10 (42.5, 100) -> (42.5, 120)
  line L11 (42.5, 120) -> (29.4185, 120)
  line L12 (29.4185, 120) -> (29.4185, 177)
  line L13 (29.4185, 177) -> (10, 177)
  line L14 (10, 177) -> (10, 180)
  line L15 (10, 180) -> (-10, 180)
  line L16 (-10, 180) -> (-10, 177)
  line L17 (-10, 177) -> (-29.4185, 177)
  line L18 (-29.4185, 177) -> (-29.4185, 120)
  line L19 (-29.4185, 120) -> (-42.5, 120)
  line L20 (-42.5, 120) -> (-42.5, 100)
  line L21 (-42.5, 100) -> (-45.5, 100)
  line L22 (-45.5, 100) -> (-45.5, 80)
  line L23 (-45.5, 80) -> (-42.5, 80)
  line L24 (-42.5, 80) -> (-42.5, 60)
  line L25 (-42.5, 60) -> (-45.5, 60)
  line L26 (-45.5, 60) -> (-45.5, 40)
  line L27 (-45.5, 40) -> (-42.5, 40)
  line L28 (-42.5, 40) -> (-42.5, 20)
  line L29 (-42.5, 20) -> (-45.5, 20)
  line L30 (-45.5, 20) -> (-45.5, 0)
  line L31 (-45.5, 0) -> (45.5, 0)
  line L32 (-39.37, 86.96) -> (39.37, 86.96)
  line L33 (0, 86.96) -> (-10, 86.96) construction
  line L34 (0, 86.96) -> (10, 86.96) construction
  line L35 (-10, 86.96) -> (-15, 86.96)
  line L36 (-15, 88.46) -> (-10, 88.46)
  line L37 (-10, 88.46) -> (-10, 86.96)
  line L38 (-15, 88.46) -> (-15, 86.96)
  line L39 (10, 86.96) -> (15, 86.96)
  line L40 (15, 86.96) -> (15, 88.46)
  line L41 (15, 88.46) -> (10, 88.46)
  line L42 (10, 88.46) -> (10, 86.96)
  line L43 (-15, 120.96) -> (-10, 120.96)
  line L44 (-10, 120.96) -> (-10, 119.46)
  line L45 (-10, 119.46) -> (-15, 119.46)
  line L46 (-15, 119.46) -> (-15, 120.96)
  line L47 (10, 120.96) -> (15, 120.96)
  line L48 (15, 120.96) -> (15, 119.46)
  line L49 (15, 119.46) -> (10, 119.46)
  line L50 (10, 119.46) -> (10, 120.96)
  dimension "d354" = 10
  dimension "d355" = 5
  dimension "d356" = 1.5
  dimension "d357" = 31
  measures "d354" distance of origin
extrude "Extrude24" cut sketch "Sketch2 (3)" against normal blind 3 contours L32 L35 L36 L37 L38 | L32 L39 L40 L41 L42 | L43 L44 L45 L46 | L47 L48 L49 L50 bodies 12 in component "MDF"
sketch "Sketch3 (2)" plane through (0, 0, 45.5) normal (0, 0, 1) x (1, 0, 0)
  line L0 (16.75, 131.5) -> (21.25, 131.5)
  line L1 (21.25, 131.5) -> (21.25, 140)
  line L2 (21.25, 140) -> (24.25, 140)
  line L3 (24.25, 140) -> (24.25, 160)
  line L4 (24.25, 160) -> (21.25, 160)
  line L5 (21.25, 160) -> (21.25, 177)
  line L6 (21.25, 177) -> (-8.1685, 177)
  line L7 (-8.1685, 177) -> (-8.1685, 120)
  line L8 (-8.1685, 120) -> (-24.25, 120)
  line L9 (-24.25, 120) -> (-24.25, 100)
  line L10 (-24.25, 100) -> (-21.25, 100)
  line L11 (-21.25, 100) -> (-21.25, 80)
  line L12 (-21.25, 80) -> (-24.25, 80)
  line L13 (-24.25, 80) -> (-24.25, 60)
  line L14 (-24.25, 60) -> (-21.25, 60)
  line L15 (-21.25, 60) -> (-21.25, 40)
  line L16 (-21.25, 40) -> (-24.25, 40)
  line L17 (-24.25, 40) -> (-24.25, 20)
  line L18 (-24.25, 20) -> (-21.25, 20)
  line L19 (-21.25, 20) -> (-21.25, 0)
  line L20 (-21.25, 0) -> (-24.25, 0)
  line L21 (-24.25, 0) -> (-24.25, -11.8717)
  arc A0 (-24.25, -11.8717) -> (24.25, -11.8717) centre (0, 0) ccw
  line L22 (24.25, -11.8717) -> (24.25, 0)
  line L23 (24.25, 0) -> (21.25, 0)
  line L24 (21.25, 0) -> (21.25, 20)
  line L25 (21.25, 20) -> (24.25, 20)
  line L26 (24.25, 20) -> (24.25, 40)
  line L27 (24.25, 40) -> (21.25, 40)
  line L28 (21.25, 40) -> (21.25, 48.5)
  line L29 (21.25, 48.5) -> (16.75, 48.5)
  line L30 (16.75, 48.5) -> (16.75, 47.15)
  line L31 (16.75, 47.15) -> (14.25, 47.15)
  line L32 (14.25, 47.15) -> (14.25, 52.85)
  line L33 (14.25, 52.85) -> (16.75, 52.85)
  line L34 (16.75, 52.85) -> (16.75, 51.5)
  line L35 (16.75, 51.5) -> (21.25, 51.5)
  line L36 (21.25, 51.5) -> (21.25, 60)
  line L37 (21.25, 60) -> (24.25, 60)
  line L38 (24.25, 60) -> (24.25, 80)
  line L39 (24.25, 80) -> (21.25, 80)
  line L40 (21.25, 80) -> (21.25, 100)
  line L41 (21.25, 100) -> (24.25, 100)
  line L42 (24.25, 100) -> (24.25, 120)
  line L43 (24.25, 120) -> (21.25, 120)
  line L44 (21.25, 120) -> (21.25, 128.5)
  line L45 (21.25, 128.5) -> (16.75, 128.5)
  line L46 (16.75, 128.5) -> (16.75, 127.15)
  line L47 (16.75, 127.15) -> (14.25, 127.15)
  line L48 (14.25, 127.15) -> (14.25, 132.85)
  line L49 (14.25, 132.85) -> (16.75, 132.85)
  line L50 (16.75, 132.85) -> (16.75, 131.5)
  circle A1 centre (0, 0) radius 11.25
  circle A2 centre (15.5, 15.5) radius 1.5
  circle A3 centre (-15.5, -15.5) radius 1.5
  circle A4 centre (15.5, -15.5) radius 1.5
  circle A5 centre (-15.5, 15.5) radius 1.5
  circle A6 centre (10.25, 54.7) radius 3
  circle A7 centre (10.25, 85.3) radius 3
  line L51 (6.25, 79.3) -> (19.25, 79.3)
  line L52 (19.25, 79.3) -> (19.25, 60.7)
  line L53 (19.25, 60.7) -> (6.25, 60.7)
  line L54 (6.25, 60.7) -> (6.25, 79.3)
  line L55 (19.25, 70) -> (24.25, 70) construction
  line L56 (10.25, 60.7) -> (10.25, 54.7) construction
  line L57 (10.25, 79.3) -> (10.25, 85.3) construction
  dimension "d363" = 6
  dimension "d364" = 6
  dimension "d365" = 18.6
  dimension "d366" = 13
  dimension "d367" = 2
  dimension "d368" = 6
  dimension "d369" = 6
  dimension "d370" = 4
  measures "d363" diameter of A6
  measures "d364" diameter of A7
  measures "d367" distance of A0.centre L52
extrude "Extrude25" cut sketch "Sketch3 (2)" against normal blind 3 contours A6 | A7 | L51 L52 L53 L54 bodies 3 in component "MDF"
sketch "Sketch4 (2)" plane through (0, 0, -42.5) normal (0, 0, 1) x (1, 0, 0)
  line L0 (16.75, 131.5) -> (21.25, 131.5)
  line L1 (21.25, 131.5) -> (21.25, 140)
  line L2 (21.25, 140) -> (24.25, 140)
  line L3 (24.25, 140) -> (24.25, 160)
  line L4 (24.25, 160) -> (21.25, 160)
  line L5 (21.25, 160) -> (21.25, 177)
  line L6 (21.25, 177) -> (-8.1685, 177)
  line L7 (-8.1685, 177) -> (-8.1685, 120)
  line L8 (-8.1685, 120) -> (-24.25, 120)
  line L9 (-24.25, 120) -> (-24.25, 100)
  line L10 (-24.25, 100) -> (-21.25, 100)
  line L11 (-21.25, 100) -> (-21.25, 80)
  line L12 (-21.25, 80) -> (-24.25, 80)
  line L13 (-24.25, 80) -> (-24.25, 60)
  line L14 (-24.25, 60) -> (-21.25, 60)
  line L15 (-21.25, 60) -> (-21.25, 40)
  line L16 (-21.25, 40) -> (-24.25, 40)
  line L17 (-24.25, 40) -> (-24.25, 20)
  line L18 (-24.25, 20) -> (-21.25, 20)
  line L19 (-21.25, 20) -> (-21.25, 0)
  line L20 (-21.25, 0) -> (-24.25, 0)
  line L21 (-24.25, 0) -> (-24.25, -11.8717)
  arc A0 (-24.25, -11.8717) -> (24.25, -11.8717) centre (0, 0) ccw
  line L22 (24.25, -11.8717) -> (24.25, 0)
  line L23 (24.25, 0) -> (21.25, 0)
  line L24 (21.25, 0) -> (21.25, 20)
  line L25 (21.25, 20) -> (24.25, 20)
  line L26 (24.25, 20) -> (24.25, 40)
  line L27 (24.25, 40) -> (21.25, 40)
  line L28 (21.25, 40) -> (21.25, 48.5)
  line L29 (21.25, 48.5) -> (16.75, 48.5)
  line L30 (16.75, 48.5) -> (16.75, 47.15)
  line L31 (16.75, 47.15) -> (14.25, 47.15)
  line L32 (14.25, 47.15) -> (14.25, 52.85)
  line L33 (14.25, 52.85) -> (16.75, 52.85)
  line L34 (16.75, 52.85) -> (16.75, 51.5)
  line L35 (16.75, 51.5) -> (21.25, 51.5)
  line L36 (21.25, 51.5) -> (21.25, 60)
  line L37 (21.25, 60) -> (24.25, 60)
  line L38 (24.25, 60) -> (24.25, 80)
  line L39 (24.25, 80) -> (21.25, 80)
  line L40 (21.25, 80) -> (21.25, 100)
  line L41 (21.25, 100) -> (24.25, 100)
  line L42 (24.25, 100) -> (24.25, 120)
  line L43 (24.25, 120) -> (21.25, 120)
  line L44 (21.25, 120) -> (21.25, 128.5)
  line L45 (21.25, 128.5) -> (16.75, 128.5)
  line L46 (16.75, 128.5) -> (16.75, 127.15)
  line L47 (16.75, 127.15) -> (14.25, 127.15)
  line L48 (14.25, 127.15) -> (14.25, 132.85)
  line L49 (14.25, 132.85) -> (16.75, 132.85)
  line L50 (16.75, 132.85) -> (16.75, 131.5)
  circle A1 centre (-15.5, 15.5) radius 1.5
  circle A2 centre (15.5, -15.5) radius 1.5
  circle A3 centre (-15.5, -15.5) radius 1.5
  circle A4 centre (15.5, 15.5) radius 1.5
  circle A5 centre (0, 0) radius 11.25
  line L51 (9.05, 86.96) -> (17.25, 86.96)
  line L52 (17.25, 86.96) -> (17.25, 68.96)
  line L53 (17.25, 68.96) -> (9.05, 68.96)
  line L54 (9.05, 68.96) -> (9.05, 86.96)
  line L55 (-18.75, 86.96) -> (-9, 86.96) construction
  dimension "d373" = 8.2
  dimension "d374" = 18
  dimension "d375" = 4
  measures "d375" distance of L40 L52
extrude "Extrude26" cut sketch "Sketch4 (2)" against normal blind 3 contours L51 L52 L53 L54 bodies 4 in component "MDF"
sketch "Sketch28" plane through (0, 0, -45.5) normal (0, 0, -1) x (-1, 0, 0) in component "MDF"
  line L0 (-17.25, 68.96) -> (-17.25, 86.96)
  line L1 (-17.25, 86.96) -> (-9.05, 86.96)
  line L2 (-9.05, 86.96) -> (-9.05, 68.96)
  line L3 (-9.05, 68.96) -> (-17.25, 68.96)
  circle A0 centre (-15.5, 15.5) radius 1.5
  circle A1 centre (15.5, -15.5) radius 1.5
  circle A2 centre (15.5, 15.5) radius 1.5
  circle A3 centre (-15.5, -15.5) radius 1.5
  circle A4 centre (0, 0) radius 11.25
  line L4 (-21.25, 131.5) -> (-16.75, 131.5)
  line L5 (-16.75, 131.5) -> (-16.75, 132.85)
  line L6 (-16.75, 132.85) -> (-14.25, 132.85)
  line L7 (-14.25, 132.85) -> (-14.25, 127.15)
  line L8 (-14.25, 127.15) -> (-16.75, 127.15)
  line L9 (-16.75, 127.15) -> (-16.75, 128.5)
  line L10 (-16.75, 128.5) -> (-21.25, 128.5)
  line L11 (-21.25, 128.5) -> (-21.25, 120)
  line L12 (-21.25, 120) -> (-24.25, 120)
  line L13 (-24.25, 120) -> (-24.25, 100)
  line L14 (-24.25, 100) -> (-21.25, 100)
  line L15 (-21.25, 100) -> (-21.25, 80)
  line L16 (-21.25, 80) -> (-24.25, 80)
  line L17 (-24.25, 80) -> (-24.25, 60)
  line L18 (-24.25, 60) -> (-21.25, 60)
  line L19 (-21.25, 60) -> (-21.25, 51.5)
  line L20 (-21.25, 51.5) -> (-16.75, 51.5)
  line L21 (-16.75, 51.5) -> (-16.75, 52.85)
  line L22 (-16.75, 52.85) -> (-14.25, 52.85)
  line L23 (-14.25, 52.85) -> (-14.25, 47.15)
  line L24 (-14.25, 47.15) -> (-16.75, 47.15)
  line L25 (-16.75, 47.15) -> (-16.75, 48.5)
  line L26 (-16.75, 48.5) -> (-21.25, 48.5)
  line L27 (-21.25, 48.5) -> (-21.25, 40)
  line L28 (-21.25, 40) -> (-24.25, 40)
  line L29 (-24.25, 40) -> (-24.25, 20)
  line L30 (-24.25, 20) -> (-21.25, 20)
  line L31 (-21.25, 20) -> (-21.25, 0)
  line L32 (-21.25, 0) -> (-24.25, 0)
  line L33 (-24.25, 0) -> (-24.25, -11.8717)
  arc A5 (-24.25, -11.8717) -> (24.25, -11.8717) centre (0, 0) ccw
  line L34 (24.25, -11.8717) -> (24.25, 0)
  line L35 (24.25, 0) -> (21.25, 0)
  line L36 (21.25, 0) -> (21.25, 20)
  line L37 (21.25, 20) -> (24.25, 20)
  line L38 (24.25, 20) -> (24.25, 40)
  line L39 (24.25, 40) -> (21.25, 40)
  line L40 (21.25, 40) -> (21.25, 60)
  line L41 (21.25, 60) -> (24.25, 60)
  line L42 (24.25, 60) -> (24.25, 80)
  line L43 (24.25, 80) -> (21.25, 80)
  line L44 (21.25, 80) -> (21.25, 100)
  line L45 (21.25, 100) -> (24.25, 100)
  line L46 (24.25, 100) -> (24.25, 120)
  line L47 (24.25, 120) -> (8.1685, 120)
  line L48 (8.1685, 120) -> (8.1685, 177)
  line L49 (8.1685, 177) -> (-21.25, 177)
  line L50 (-21.25, 177) -> (-21.25, 160)
  line L51 (-21.25, 160) -> (-24.25, 160)
  line L52 (-24.25, 160) -> (-24.25, 140)
  line L53 (-24.25, 140) -> (-21.25, 140)
  line L54 (-21.25, 140) -> (-21.25, 131.5)
  line L55 (0, 0) -> (3, 0)
  line L56 (3, 0) -> (0, 0)
  line L57 (0, 0) -> (-3, 0)
  line L58 (3, 0) -> (3, -30)
  line L59 (3, -30) -> (-3, -30)
  line L60 (-3, -30) -> (-3, 0)
  dimension "d378" = 3
  dimension "d379" = 3
  dimension "d380" = 30
  measures "d378" distance of A4.centre
  measures "d379" distance of A4.centre
extrude "Extrude27" cut sketch "Sketch28" against normal blind 130 contours A4 L55 L56 L57 L58 L60 | A4 A5 L58 L60 | A5 L58 L59 L60 picked at (2, -3.6142) bodies 3 4 in component "MDF"
fillet "Fillet1'" radius 2 12 edges at (3, -10.8426, 44) (-3, -26.8328, 44) (3, -26.8328, 44) (-3, -10.8426, 44) (24.25, -11.8717, 44) (-24.25, -11.8717, 44) (3, -10.8426, -44) (3, -26.8328, -44) (-3, -26.8328, -44) (-3, -10.8426, -44) (24.25, -11.8717, -44) (-24.25, -11.8717, -44) on bodies 3 4 in component "MDF"
component "Steppers" placed x (1, 0, 0) y (0, 1, 0) z (0, 0, 1) at (0, 0, 0)
component "MDF" placed x (1, 0, 0) y (0, 1, 0) z (0, 0, 1) at (0, 0, 0)
component "Wheels" placed x (1, 0, 0) y (0, 1, 0) z (0, 0, 1) at (0, 0, 0)
component "ground plane" placed x (1, 0, 0) y (0, 1, 0) z (0, 0, 1) at (0, 0, 0)
component "pcb" placed x (1, 0, 0) y (0, 1, 0) z (0, 0, 1) at (0, 0, 0)
equation "d3 = d28 / 2"
equation "d4 = d28 / 2"
equation "d9 = ( 31 / 2 ) * 1 mm"
equation "d10 = d9"
equation "d11 = d9"
equation "d12 = d9"
equation "d13 = d9"
equation "d14 = d9"
equation "d15 = d9"
equation "d16 = d9"
equation "d29 = d28"
equation "d31 = d30"
equation "d32 = d30"
equation "d33 = d30"
equation "thick = 3 mm"
equation "d38 = thick"
equation "d39 = thick"
equation "d42 = thick"
equation "d46 = -85 mm - thick"
equation "d48 = thick - 2.5 mm"
equation "wheelDia = 88 mm"
equation "d56 = wheelDia"
equation "d69 = thick"
equation "d71 = thick"
equation "d73 = thick"
equation "d75 = thick"
equation "d77 = thick"
equation "d79 = thick"
equation "d82 = thick"
equation "d84 = thick"
equation "d86 = thick"
equation "d88 = thick"
equation "d90 = thick"
equation "d92 = thick"
equation "d94 = -thick"
equation "d99 = thick"
equation "d101 = thick"
equation "d102 = thick"
equation "d104 = thick"
equation "d105 = thick"
equation "d109 = thick"
equation "d110 = thick"
equation "d196 = 42.5 mm + thick"
equation "d248 = thick"
equation "d249 = thick"
equation "d253 = thick"
equation "d257 = ( ( 41.4 - 16 ) / 2 ) * 1 mm"
equation "d258 = d257"
equation "d261 = -thick"
equation "d263 = ( ( 41.4 - 16 ) / 2 ) * 1 mm"
equation "d264 = d263"
equation "d267 = -thick"
equation "d269 = -thick"
equation "d271 = -thick"
equation "d273 = -thick"
equation "d275 = -thick"
equation "d277 = ( ( 41.4 - 16 ) / 2 ) * 1 mm"
equation "d278 = d277"
equation "d281 = -thick"
equation "d291 = ( 78.74 / 2 ) * 1 mm"
equation "d300 = ( 43.18 / 2 ) * 1 mm"
equation "d316 = d315"
equation "d318 = d317"
equation "d320 = d319"
equation "d324 = d323"
equation "d331 = -thick"
equation "d334 = ( 3 / 2 ) * 1 mm"
equation "d336 = 10 mm - thick"
equation "d338 = ( 5.7 / 2 ) * 1 mm"
equation "d340 = ( 3 / 2 ) * 1 mm"
equation "d342 = 10 mm - thick"
equation "d344 = ( 5.7 / 2 ) * 1 mm"
equation "d351 = -thick"
equation "d358 = -thick"
equation "d371 = -thick"
equation "d376 = -thick"
